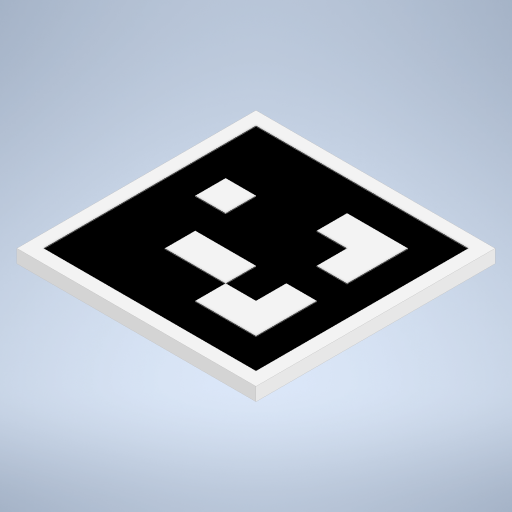
# Autodesk Inventor part: marker_base
Saved by Autodesk Inventor 2024.1 (Build 281209000, 209)
## iProperties
Created: 2025-06-23
Part Number: marker_base
Material: 一般
Document SubType Name: Modeling
Designer: hibik
Density: 1 g/cm^3
Appearance: 既定
Author: hibik
Autodesk Inventor part; units mm, degrees
ref_plane "YZ Plane" through (0, 0, 0) normal (1, 0, 0) x (0, 1, 0)
ref_plane "XZ Plane" through (0, 0, 0) normal (0, 1, 0) x (-1, 0, 0)
ref_plane "XY Plane" through (0, 0, 0) normal (0, 0, 1) x (1, 0, 0)
sketch "スケッチ1" plane through (0, 0, 0) normal (0, 1, 0) x (-1, 0, 0)
  line L0 (16, 16) -> (-16, 16)
  line L1 (-16, 16) -> (-16, -16)
  line L2 (-16, -16) -> (16, -16)
  line L3 (16, -16) -> (16, 16)
  line L4 (16, 16) -> (-16, -16) construction
  line L5 (-16, 16) -> (16, -16) construction
  line L6 (18, 18) -> (-18, 18)
  line L7 (-18, 18) -> (-18, -18)
  line L8 (-18, -18) -> (18, -18)
  line L9 (18, -18) -> (18, 18)
  line L10 (18, 18) -> (-18, -18) construction
  line L11 (-18, 18) -> (18, -18) construction
  line L12 (2.2857, 16) -> (2.2857, -16)
  line L13 (6.8571, 16) -> (6.8571, -16)
  line L14 (11.4286, 16) -> (11.4286, -16)
  line L15 (0, -25.2) -> (0, 25.2) construction
  line L16 (25.2, 0) -> (-25.2, 0) construction
  line L17 (-2.2857, 16) -> (-2.2857, -16)
  line L18 (-6.8571, 16) -> (-6.8571, -16)
  line L19 (-11.4286, 16) -> (-11.4286, -16)
  line L20 (16, 11.4286) -> (-16, 11.4286)
  line L21 (16, 6.8576) -> (-16, 6.8576)
  line L22 (16, 2.2866) -> (-16, 2.2866)
  line L23 (16, -2.2844) -> (-16, -2.2844)
  line L24 (16, -6.8554) -> (-16, -6.8554)
  line L25 (16, -11.4264) -> (-16, -11.4264)
  point P0 (0, 0)
  point P1 (0, 16)
  point P2 (-11.4286, 2.2866)
  point P3 (-6.8571, 2.2866)
  point P4 (-6.8571, 6.8576)
  point P5 (-11.4286, 6.8576)
  point P6 (-2.2857, -6.8554)
  point P7 (-2.2857, -2.2844)
  point P8 (-11.4286, -2.2844)
  point P9 (-11.4286, -11.4264)
  point P10 (2.2857, -11.4264)
  point P11 (2.2857, -6.8554)
  point P12 (11.4286, 6.8576)
  point P13 (6.8571, 6.8576)
  point P14 (6.8571, 2.2866)
  point P15 (-2.2857, 2.2866)
  point P16 (6.8571, -2.2844)
  point P17 (6.8571, -6.8554)
  point P18 (11.4286, -6.8554)
  point P19 (2.2857, -2.2844)
  point P20 (-6.8571, -11.4264)
  point P21 (-2.2857, -11.4264)
  point P22 (-6.8571, -6.8554)
  point P23 (-11.4286, -6.8554)
  point P24 (-6.8571, -2.2844)
  point P25 (-6.8571, 11.4286)
  point P26 (-11.4286, 11.4286)
  point P27 (11.4286, 11.4286)
  point P28 (-2.2857, 11.4286)
  point P29 (-2.2857, 6.8576)
  point P30 (11.4286, -2.2844)
  dimension "d0" = 32
  dimension "d1" = 32
  dimension "d2" = 36
  dimension "d3" = 36
  dimension "d4" = 4.5714
  dimension "d5" = 4.5714
  dimension "d6" = 4.5714
  dimension "d7" = 2.2857
  dimension "d8" = 4.5714
  dimension "d18" = 4.571
  constraints: 48 end point, 8 point on line, 6 perpendicular, 6 symmetric about line, 5 midpoint, 4 parallel, 2 horizontal, 1 vertical, 15 other
  measures "d0" distance of L2.end L1.end
  measures "d1" distance of L1.end L0.end
  measures "d2" distance of L8.end L7.end
  measures "d3" distance of L7.end L6.end
  measures "d4" distance between parallel lines of L3 L14
  measures "d5" distance between parallel lines of L13 L14
  measures "d6" distance between parallel lines of L13 L12
  measures "d7" distance from line of point (0, 16) L12
  measures "d8" distance between parallel lines of L20 L0
  measures "d18" distance of L20.start L21.start
extrude "押し出し1" add sketch "スケッチ1" along normal blind 2 contours L13 L22 L12 L21 | L17 L21 L18 L20 | L12 L22 L17 L21 | L14 L24 L13 L23 | L18 L21 L19 L20 | L18 L22 L19 L21 | L18 L24 L19 L23 | L17 L25 L18 L24 | L18 L25 L19 L24 | L9 L8 L7 L6
sketch "スケッチ2" plane through (0, 0, 0) normal (0, -1, 0) x (1, 0, 0)
  line L0 (-18, -18) -> (-18, 18) projected
  line L1 (-18, 18) -> (18, 18) projected
  line L2 (-18, -18) -> (18, -18)
  line L3 (18, -18) -> (18, 18)
  line L4 (18, 18) -> (-18, 18)
  line L5 (-18, 18) -> (-18, -18)
  point P0 (0, 0)
  constraints: 8 end point, 2 parallel, 1 horizontal, 1 perpendicular
extrude "押し出し2" add sketch "スケッチ2" against normal blind 1.9
equation "\"d4\" = 2 * d7"
equation "\"d5\" = d4"
equation "\"d6\" = d5"
equation "\"d8\" = d4"
